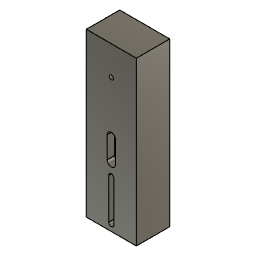
Seitenhalterung für mitte rechts v2 (Autodesk Fusion 360 design; units mm, degrees)
Autodesk Fusion 360 part; units mm, degrees
sketch "Skizze1" plane through (0, 0, 0) normal (0, 0, 1) x (1, 0, 0)
  line L0 (30, 20) -> (-30, 20)
  line L1 (-30, 20) -> (-30, -20)
  line L2 (-30, -20) -> (30, -20)
  line L3 (30, -20) -> (30, 20)
  line L4 (30, 20) -> (-30, -20) construction
  line L5 (-30, 20) -> (30, -20) construction
  dimension "d2" = 60
  dimension "d3" = 40
  constraint perpendicular L0 L1
  constraint parallel L0 L2
  constraint parallel L1 L3
  constraint horizontal L0
  constraint coincident L4 origin
  constraint coincident L5 origin
  measures "d2" distance of L1.end L2.end
  measures "d3" distance of L0.end L1.end
extrude "Extrusion1" add sketch "Skizze1" along normal blind 195 makes body 1
sketch "Skizze3" plane through (0, -20, 0) normal (0, -1, 0) x (1, 0, 0)
  line L0 (-30, 0) -> (30, 0)
  line L1 (30, 0) -> (30, 195)
  line L2 (30, 195) -> (-30, 195)
  line L3 (-30, 195) -> (-30, 0)
  line L4 (3.1, 8.1) -> (3.1, 56.9)
  arc A0 (3.1, 56.9) -> (-3.1, 56.9) centre (0, 56.9) ccw
  line L5 (-3.1, 56.9) -> (-3.1, 8.1)
  arc A1 (-3.1, 8.1) -> (3.1, 8.1) centre (0, 8.1) ccw
  line L6 (0, 5) -> (0, 60) construction
  line L7 (2.5, 72.5) -> (2.5, 97.5)
  arc A2 (2.5, 97.5) -> (-2.5, 97.5) centre (0, 97.5) ccw
  line L8 (-2.5, 97.5) -> (-2.5, 72.5)
  arc A3 (-2.5, 72.5) -> (2.5, 72.5) centre (0, 72.5) ccw
  line L9 (0, 70) -> (0, 100) construction
  point P0 (0, 195)
  dimension "d20" = 6.2
  dimension "d21" = 5
  constraint midpoint L2 P0
  constraint tangent L4 A0
  constraint tangent A0 L5
  constraint parallel L4 L5
  constraint tangent L5 A1
  constraint tangent L4 A1
  constraint midpoint A1 L6.start
  constraint midpoint A0 L6.end
  constraint parallel L3 L6
  constraint tangent L7 A2
  constraint tangent A2 L8
  constraint parallel L7 L8
  constraint tangent L8 A3
  constraint tangent L7 A3
  constraint midpoint A3 L9.start
  constraint midpoint A2 L9.end
  constraint parallel L6 L9
  measures "d20" diameter of A0
  measures "d21" diameter of A2
extrude "Extrusion2" cut sketch "Skizze3" against normal blind 40 contours L4 A0 L5 A1 | L7 A2 L8 A3 bodies 1
sketch "Skizze4" plane through (30, 0, 0) normal (1, 0, 0) x (0, 1, 0)
  line L0 (-20, 0) -> (20, 0)
  line L1 (20, 0) -> (20, 195)
  line L2 (20, 195) -> (-20, 195)
  line L3 (-20, 195) -> (-20, 0)
  circle A0 centre (0, 174.5) radius 4.15
  dimension "d12" = 8.3
  measures "d12" diameter of A0
extrude "Extrusion3" add sketch "Skizze4" against normal blind 60 separate body contours A0 makes body 2
sketch "Skizze6" plane through (0, 0, 0) normal (0, 1, 0) x (1, 0, 0)
sketch "Skizze7" plane through (0, 20, 0) normal (0, 1, 0) x (-1, 0, 0)
  line L0 (-30, 0) -> (30, 0)
  line L1 (30, 0) -> (30, 195)
  line L2 (30, 195) -> (-30, 195)
  line L3 (-30, 195) -> (-30, 0)
  circle A0 centre (0, 160) radius 2.5
  line L4 (-2.5, 72.5) -> (-2.5, 97.5)
  arc A1 (2.5, 97.5) -> (-2.5, 97.5) centre (0, 97.5) ccw
  line L5 (2.5, 97.5) -> (2.5, 72.5)
  arc A2 (-2.5, 72.5) -> (2.5, 72.5) centre (0, 72.5) ccw
  line L6 (-3.1, 8.1) -> (-3.1, 56.9)
  arc A3 (3.1, 56.9) -> (-3.1, 56.9) centre (0, 56.9) ccw
  line L7 (3.1, 56.9) -> (3.1, 8.1)
  arc A4 (-3.1, 8.1) -> (3.1, 8.1) centre (0, 8.1) ccw
  dimension "d17" = 5
  measures "d17" diameter of A0
extrude "Extrusion4" cut sketch "Skizze7" against normal blind 40 contours A0 bodies 1
sketch "Skizze8" plane through (0, -20, 0) normal (0, -1, 0) x (1, 0, 0)
  circle A0 centre (0, 160) radius 2.5
  line L0 (2.5, 97.5) -> (2.5, 72.5)
  arc A1 (-2.5, 72.5) -> (2.5, 72.5) centre (0, 72.5) ccw
  line L1 (-2.5, 72.5) -> (-2.5, 97.5)
  arc A2 (2.5, 97.5) -> (-2.5, 97.5) centre (0, 97.5) ccw
  line L2 (3.1, 56.9) -> (3.1, 8.1)
  arc A3 (-3.1, 8.1) -> (3.1, 8.1) centre (0, 8.1) ccw
  line L3 (-3.1, 8.1) -> (-3.1, 56.9)
  arc A4 (3.1, 56.9) -> (-3.1, 56.9) centre (0, 56.9) ccw
  line L4 (-30, 0) -> (30, 0)
  line L5 (30, 0) -> (30, 195)
  line L6 (30, 195) -> (-30, 195)
  line L7 (-30, 195) -> (-30, 0)
  line L8 (5, 72) -> (5, 98)
  arc A5 (5, 98) -> (-5, 98) centre (0, 98) ccw
  line L9 (-5, 98) -> (-5, 72)
  arc A6 (-5, 72) -> (5, 72) centre (0, 72) ccw
  line L10 (0, 72) -> (0, 98) construction
  constraint tangent L8 A5
  constraint tangent A5 L9
  constraint parallel L8 L9
  constraint tangent L9 A6
  constraint tangent L8 A6
  constraint vertical L10
extrude "Extrusion5" cut sketch "Skizze8" against normal blind 9 contours L8 A5 L9 A6 bodies 1
extrude "Extrusion7" cut 1 faces at (-30, -1.0141, 173.1467) along direction (1, 0, 0) blind 50 on bodies 2 bodies 1 2
combine "Kombinieren2" operation add target body 1 tool bodies 2
